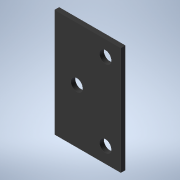
# Autodesk Inventor part: hinge flag plate
Saved by Autodesk Inventor 2020 (Build 240168000, 168)
## iProperties
Created: 2023-04-24
Part Number: hinge flag plate
Material: Generic
Document SubType Name: Modeling
Designer: super
Density: 1 g/cm^3
Appearance: Default
Author: super
Autodesk Inventor part; units mm, degrees
ref_plane "YZ Plane" through (0, 0, 0) normal (1, 0, 0) x (0, 1, 0)
ref_plane "XZ Plane" through (0, 0, 0) normal (0, 1, 0) x (-1, 0, 0)
ref_plane "XY Plane" through (0, 0, 0) normal (0, 0, 1) x (1, 0, 0)
sketch "Sketch1" plane through (0, 0, 0) normal (0, 0, 1) x (1, 0, 0)
  line L0 (0, 0) -> (30, 0)
  line L1 (30, 0) -> (30, 49)
  line L2 (30, 49) -> (0, 49)
  line L3 (0, 49) -> (0, 0)
  circle A0 centre (23, 42) radius 2.75
  circle A1 centre (10, 24.5) radius 2.75
  circle A2 centre (23, 7) radius 2.75
  dimension "d0" = 30
  dimension "d1" = 49
  dimension "d2" = 5.5
  dimension "d3" = 7
  dimension "d4" = 7
  dimension "d5" = 5.5
  dimension "d6" = 24.5
  dimension "d7" = 10
  constraints: 8 end point, 3 centre point, 2 parallel, 1 horizontal, 1 perpendicular
  measures "d0" distance of L1.end L2.end
  measures "d1" distance of L0.end L1.end
  measures "d2" diameter of A0
  measures "d3" horizontal distance of A0.centre L1.end
  measures "d4" horizontal distance of L1.end A0.centre
  measures "d5" diameter of A1
  measures "d6" vertical distance of A1.centre L2.end
  measures "d7" horizontal distance of A1.centre L2.end
extrude "Extrusion1" add sketch "Sketch1" along normal blind 2
body "Solid1"
